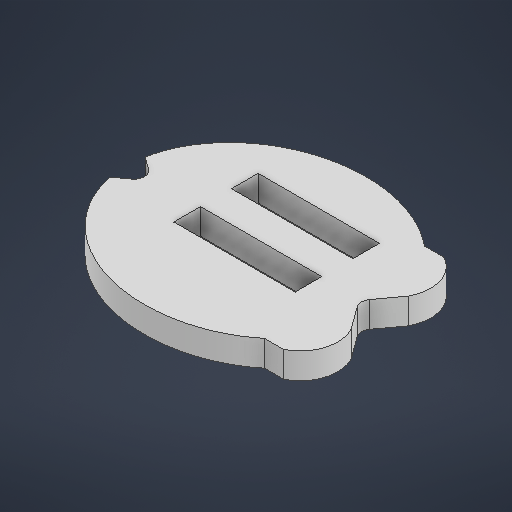
# Autodesk Inventor part: telapak kaki
Saved by Autodesk Inventor 2026.2 (Build 302298010, 298A)
## iProperties
Created: 2026-05-10
Part Number: telapak kaki
Material: Generic
Document SubType Name: Modeling
Designer: Martina
Density: 1 g/cm^3
Appearance: Default
Author: Martina
Autodesk Inventor part; units mm, degrees
ref_plane "YZ Plane" through (0, 0, 0) normal (1, 0, 0) x (0, 1, 0)
ref_plane "XZ Plane" through (0, 0, 0) normal (0, 1, 0) x (-1, 0, 0)
ref_plane "XY Plane" through (0, 0, 0) normal (0, 0, 1) x (1, 0, 0)
sketch "Sketch1" plane through (0, 0, 0) normal (0, 1, 0) x (-1, 0, 0)
  line L0 (0, 0) -> (90, 0)
  line L1 (90, 0) -> (90, -55.8)
  line L2 (90, -55.8) -> (0, -55.8)
  line L3 (0, -55.8) -> (0, 0)
  ellipse E0 centre (45, -27.9) end of major axis (0, -27.9) minor radius 38.6219 (13.883, -55.8) -> (13.883, 0) ccw
  line L4 (64.8234, -39.45) -> (22.5234, -39.45)
  line L5 (22.5234, -39.45) -> (22.5234, -48.75)
  line L6 (22.5234, -48.75) -> (64.8234, -48.75)
  line L7 (64.8234, -48.75) -> (64.8234, -39.45)
  line L8 (64.8234, -19.35) -> (22.5234, -19.35)
  line L9 (22.5234, -19.35) -> (22.5234, -28.65)
  line L10 (22.5234, -28.65) -> (64.8234, -28.65)
  line L11 (64.8234, -28.65) -> (64.8234, -19.35)
  line L12 (90, -27.9) -> (0, -27.9)
  ellipse E1 centre (12.4971, -44.1) end of major axis (0, -44.1) minor radius 12.8946 (3.6964, -34.945) -> (15.0472, -56.7233) ccw
  line L13 (1.5364, -17.8943) -> (7.2883, -25.7782)
  line L14 (1.5364, -37.9057) -> (7.2883, -30.0218)
  arc A0 (7.2883, -30.0218) -> (7.2883, -25.7782) centre (4.38, -27.9) ccw
  line L15 (85.0982, -24.9854) -> (89.4419, -21.8362)
  line L16 (85.0982, -30.8146) -> (89.4419, -33.9638)
  arc A1 (85.0982, -24.9854) -> (85.0982, -30.8146) centre (87.2113, -27.9) ccw
  ellipse E2 centre (12.4971, -11.7) end of major axis (0, -11.7) minor radius 12.8946 (15.0472, 0.9233) -> (3.6964, -20.855) ccw
  ellipse E3 centre (12.4971, -11.7) end of major axis (0, -11.7) minor radius 12.8946 (22.5234, -19.3972) -> (22.5573, -19.35) ccw
  point P0 (8.8363, -27.9)
  point P1 (81.0782, -27.9)
  point P2 (7.2438, 0)
  point P3 (7.2438, -55.8)
  dimension "d0" = 90
  dimension "d1" = 55.8
  dimension "d3" = 9.3
  dimension "d4" = 9.3
  dimension "d5" = 7.05
  dimension "d6" = 10.8
  dimension "d7" = 3.6
  dimension "d8" = 3.6
  constraints: 34 end point, 14 point on line, 6 parallel, 4 point on circle, 4 tangent, 3 horizontal, 3 perpendicular, 2 centre point, 2 midpoint, 2 symmetric about line, 1 vertical, 21 other
  measures "d0" distance of L1.end L2.end
  measures "d1" distance of L0.end L1.end
  measures "d3" distance of L5.end L4.end
  measures "d4" distance of L9.end L8.end
  measures "d5" distance between parallel lines of L6 L2
  measures "d6" distance between parallel lines of L10 L4
  measures "d7" radius of A0
  measures "d8" radius of A1
extrude "Extrusion1" add sketch "Sketch1" along normal blind 9 contours L0 E0 L15 A1 L12 L11 L8 L9 A0 L13 E2 | E0 L0 | E1 L14 A0 L12 L9 L10 L11 A1 L16 E0 L2 | L2 E0
body "Solid1"
